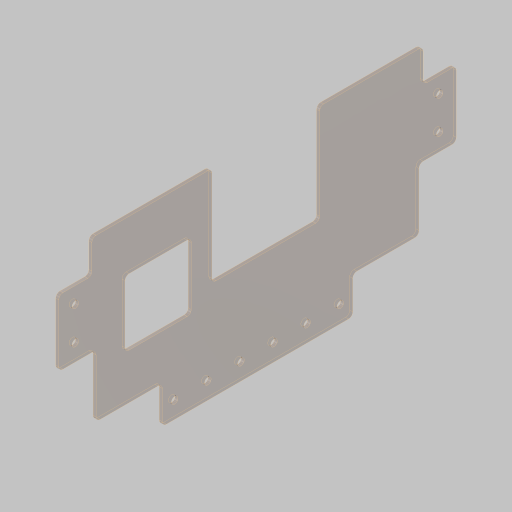
# Autodesk Inventor part: DB1-025
Saved by Autodesk Inventor 2023.5 (Build 275446000, 446)
## iProperties
Created: 2025-03-10
Part Number: DB1-025
Material: Polycarbonate, Smoke
Document SubType Name: Modeling
Designer: brand
Density: 1.2 g/cm^3
Appearance: Polycarbonate - Smoked
Author: brand
Autodesk Inventor part; units mm, degrees
ref_plane "YZ Plane" through (0, 0, 0) normal (1, 0, 0) x (0, 1, 0)
ref_plane "XZ Plane" through (0, 0, 0) normal (0, 1, 0) x (-1, 0, 0)
ref_plane "XY Plane" through (0, 0, 0) normal (0, 0, 1) x (1, 0, 0)
sketch "Sketch1" plane through (0, 0, 0) normal (1, 0, 0) x (0, 1, 0)
  line L0 (76.2, 152.4) -> (-76.2, 152.4)
  line L1 (-76.2, 152.4) -> (-76.2, -152.4)
  line L2 (-76.2, -152.4) -> (76.2, -152.4)
  line L3 (76.2, -152.4) -> (76.2, 152.4)
  line L4 (76.2, 152.4) -> (-76.2, -152.4) construction
  line L5 (-76.2, 152.4) -> (76.2, -152.4) construction
  line L6 (38.1, 101.6) -> (-12.7, 101.6)
  line L7 (-12.7, 101.6) -> (-12.7, 50.8)
  line L8 (-12.7, 50.8) -> (38.1, 50.8)
  line L9 (38.1, 50.8) -> (38.1, 101.6)
  line L10 (38.1, 101.6) -> (-12.7, 50.8) construction
  line L11 (-12.7, 101.6) -> (38.1, 50.8) construction
  line L12 (76.2, 34.925) -> (0, 34.925)
  line L13 (0, 34.925) -> (0, -47.625)
  line L14 (0, -47.625) -> (76.2, -47.625)
  line L15 (76.2, -47.625) -> (76.2, 34.925)
  line L16 (76.2, 34.925) -> (0, -47.625) construction
  line L17 (0, 34.925) -> (76.2, -47.625) construction
  point P0 (0, 0)
  point P1 (12.7, 76.2)
  point P2 (38.1, -6.35)
  point P3 (76.2, -6.35)
  point P4 (76.2, 0)
  point P5 (76.2, -47.625)
  point P6 (0, 44.45)
  point P7 (31.75, 44.45)
  point P8 (76.2, 34.925)
  dimension "d0" = 152.4
  dimension "d1" = 304.8
  dimension "d2" = 50.8
  dimension "d3" = 88.9
  dimension "d4" = 76.2
  dimension "d39" = 76.2
  dimension "d40" = 82.55
  dimension "d41" = 146.05
  constraints: 36 end point, 8 midpoint, 6 parallel, 4 perpendicular, 3 horizontal, 1 collinear
  measures "d0" distance of L2.end L1.end
  measures "d1" distance of L1.end L0.end
  measures "d2" distance of L8.end L6.start
  measures "d3" distance from line of L1 point (12.7, 76.2)
  measures "d4" distance from line of point (12.7, 76.2) L0
  measures "d39" distance of L13.end L14.end
  measures "d40" distance between parallel lines of L14 L12
  measures "d41" distance from line of L2 point (38.1, -6.35)
extrude "Extrusion1" add sketch "Sketch1" along normal blind 2.286 contours L3 L12 L13 L14 L2 L1 L0
fillet "Fillet1" radius 3.175 8 edges at (1.143, 38.1, 50.8) (1.143, 38.1, 101.6) (1.143, -12.7, 101.6) (1.143, -12.7, 50.8) (1.143, 76.2, 152.4) (1.143, 76.2, -152.4) (1.143, -76.2, -152.4) (1.143, -76.2, 152.4)
sketch "Sketch2" plane through (2.286, 0, 0) normal (1, 0, 0) x (0, 0, -1)
  arc A0 (-152.4, -73.025) -> (-149.225, -76.2) centre (-149.225, -73.025) ccw construction
  line L0 (-152.4, -73.025) -> (-152.4, 73.025) construction
  arc A1 (-149.225, 76.2) -> (-152.4, 73.025) centre (-149.225, 73.025) ccw construction
  line L1 (-149.225, 76.2) -> (-34.925, 76.2) construction
  arc A2 (152.4, 73.025) -> (149.225, 76.2) centre (149.225, 73.025) ccw construction
  line L2 (152.4, 73.025) -> (152.4, -73.025) construction
  arc A3 (149.225, -76.2) -> (152.4, -73.025) centre (149.225, -73.025) ccw construction
  line L3 (149.225, -76.2) -> (-149.225, -76.2) construction
  line L4 (-34.925, 76.2) -> (-34.925, 0) projected
  line L5 (-34.925, 0) -> (47.625, 0) projected
  line L6 (47.625, 0) -> (47.625, 76.2) projected
  line L7 (47.625, 76.2) -> (149.225, 76.2) projected
  arc A4 (-53.975, -12.7) -> (-50.8, -9.525) centre (-53.975, -9.525) ccw projected
  line L8 (-50.8, -9.525) -> (-50.8, 34.925) projected
  arc A5 (-50.8, 34.925) -> (-53.975, 38.1) centre (-53.975, 34.925) ccw projected
  line L9 (-53.975, 38.1) -> (-98.425, 38.1) projected
  arc A6 (-98.425, 38.1) -> (-101.6, 34.925) centre (-98.425, 34.925) ccw projected
  line L10 (-101.6, 34.925) -> (-101.6, -9.525) projected
  arc A7 (-101.6, -9.525) -> (-98.425, -12.7) centre (-98.425, -9.525) ccw projected
  line L11 (-98.425, -12.7) -> (-53.975, -12.7) projected
  point P0 (0, 0)
  point P1 (-139.7, -63.5)
  point P2 (139.7, -63.5)
  point P3 (-139.7, -38.1)
  point P4 (139.7, -38.1)
  point P5 (-139.7, -12.7)
  point P6 (139.7, -12.7)
  point P7 (-139.7, 12.7)
  point P8 (139.7, 12.7)
  point P9 (-139.7, 38.1)
  point P10 (139.7, 38.1)
  point P11 (-139.7, 63.5)
  point P12 (139.7, 63.5)
  point P13 (-114.3, -63.5)
  point P14 (-88.9, -63.5)
  point P15 (-63.5, -63.5)
  point P16 (-38.1, -63.5)
  point P17 (-12.7, -63.5)
  point P18 (12.7, -63.5)
  point P19 (38.1, -63.5)
  point P20 (63.5, -63.5)
  point P21 (88.9, -63.5)
  point P22 (114.3, -63.5)
  point P23 (139.7, -63.5)
  dimension "d8" = 12.7
  dimension "d9" = 12.7
  dimension "d10" = 12.7
  dimension "d13" = 25.4
  dimension "d34" = 25.4
  constraints: 1 horizontal, 1 horizontal alignment, 1 vertical, 21 other
  measures "d8" distance from line of L0 point (-139.7, -63.5)
  measures "d9" distance from line of L2 point (139.7, -63.5)
  measures "d10" distance from line of L3 point (139.7, -63.5)
  measures "d13" distance of point (-139.7, -63.5) point (-139.7, -38.1)
  measures "d34" distance of point (-139.7, -63.5) point (-114.3, -63.5)
hole "Hole1" at (2.286, -63.5, 139.7) at (2.286, -63.5, -139.7) at (2.286, -38.1, 139.7) at (2.286, -38.1, -139.7) at (2.286, -12.7, 139.7) at (2.286, -12.7, -139.7) at (2.286, 12.7, 139.7) at (2.286, 12.7, -139.7) at (2.286, 38.1, 139.7) at (2.286, 38.1, -139.7) at (2.286, 63.5, 139.7) at (2.286, 63.5, -139.7) at (2.286, -63.5, 88.9) at (2.286, -63.5, 63.5) at (2.286, -63.5, 38.1) at (2.286, -63.5, 12.7) at (2.286, -63.5, -12.7) at (2.286, -63.5, -38.1) at (2.286, -63.5, -63.5) at (2.286, -63.5, -88.9) direction (-1, 0, 0) diameter 5.1054 end through all clearance for "Flat Head Machine Screw (82)" size "#10" standard "Ansi Unified Screw Threads"
sketch "Sketch3" plane through (2.286, 0, 0) normal (1, 0, 0) x (0, 0, -1)
  line L0 (-123.825, 0) -> (-152.4, 0)
  line L1 (-152.4, 0) -> (-152.4, -76.2)
  line L2 (-152.4, -76.2) -> (-123.825, -76.2)
  line L3 (-123.825, -76.2) -> (-123.825, 0)
  line L4 (-123.825, 0) -> (-152.4, -76.2) construction
  line L5 (-152.4, 0) -> (-123.825, -76.2) construction
  circle A0 centre (-139.7, 63.5) radius 2.5527 construction
  circle A1 centre (-139.7, 38.1) radius 2.5527 construction
  circle A2 centre (-139.7, 12.7) radius 2.5527 construction
  circle A3 centre (-139.7, -12.7) radius 2.5527 construction
  circle A4 centre (-139.7, -38.1) radius 2.5527 construction
  circle A5 centre (-139.7, -63.5) radius 2.5527 construction
  circle A6 centre (139.7, -63.5) radius 2.5527 construction
  circle A7 centre (139.7, -38.1) radius 2.5527 construction
  circle A8 centre (139.7, -12.7) radius 2.5527 construction
  circle A9 centre (139.7, 12.7) radius 2.5527 construction
  circle A10 centre (139.7, 38.1) radius 2.5527 construction
  circle A11 centre (139.7, 63.5) radius 2.5527 construction
  arc A12 (-152.4, -73.025) -> (-149.225, -76.2) centre (-149.225, -73.025) ccw construction
  line L6 (-152.4, -73.025) -> (-152.4, 73.025) construction
  arc A13 (-149.225, 76.2) -> (-152.4, 73.025) centre (-149.225, 73.025) ccw construction
  line L7 (-149.225, 76.2) -> (-34.925, 76.2) construction
  arc A14 (152.4, 73.025) -> (149.225, 76.2) centre (149.225, 73.025) ccw construction
  line L8 (152.4, 73.025) -> (152.4, -73.025) construction
  arc A15 (149.225, -76.2) -> (152.4, -73.025) centre (149.225, -73.025) ccw construction
  line L9 (149.225, -76.2) -> (-149.225, -76.2) construction
  line L10 (-149.225, -76.2) -> (149.225, -76.2) construction
  line L11 (149.225, 76.2) -> (-149.225, 76.2) construction
  line L12 (0, 76.2) -> (0, -76.2) construction
  line L13 (-149.225, -76.2) -> (149.225, -76.2) construction
  line L14 (-152.4, -47.625) -> (-73.025, -47.625)
  line L15 (-73.025, -47.625) -> (-73.025, -76.2)
  line L16 (-73.025, -76.2) -> (-152.4, -76.2)
  line L17 (-152.4, -76.2) -> (-152.4, -47.625)
  line L18 (-152.4, -47.625) -> (-73.025, -76.2) construction
  line L19 (-73.025, -47.625) -> (-152.4, -76.2) construction
  line L20 (123.825, 0) -> (152.4, 0)
  line L21 (152.4, 0) -> (152.4, -76.2)
  line L22 (152.4, -76.2) -> (123.825, -76.2)
  line L23 (123.825, -76.2) -> (123.825, 0)
  line L24 (123.825, 0) -> (152.4, -76.2) construction
  line L25 (152.4, 0) -> (123.825, -76.2) construction
  circle A16 centre (139.7, -12.7) radius 2.5527 construction
  circle A17 centre (139.7, -38.1) radius 2.5527 construction
  circle A18 centre (139.7, -63.5) radius 2.5527 construction
  arc A19 (149.225, -76.2) -> (152.4, -73.025) centre (149.225, -73.025) ccw construction
  arc A20 (98.425, -25.4) -> (101.6, -22.225) centre (98.425, -22.225) ccw construction
  line L26 (152.4, -47.625) -> (73.025, -47.625)
  line L27 (73.025, -47.625) -> (73.025, -76.2)
  line L28 (73.025, -76.2) -> (152.4, -76.2)
  line L29 (152.4, -76.2) -> (152.4, -47.625)
  line L30 (152.4, -47.625) -> (73.025, -76.2) construction
  line L31 (73.025, -47.625) -> (152.4, -76.2) construction
  circle A21 centre (63.5, -63.5) radius 2.5527 projected
  circle A22 centre (12.7, -63.5) radius 2.5527 projected
  circle A23 centre (-38.1, -63.5) radius 2.5527 projected
  circle A24 centre (-88.9, -63.5) radius 2.5527 projected
  circle A25 centre (-63.5, -63.5) radius 2.5527 projected
  circle A26 centre (-12.7, -63.5) radius 2.5527 projected
  circle A27 centre (38.1, -63.5) radius 2.5527 projected
  circle A28 centre (88.9, -63.5) radius 2.5527 projected
  line L32 (-34.925, 76.2) -> (-34.925, 0) projected
  line L33 (-34.925, 0) -> (47.625, 0) projected
  line L34 (47.625, 0) -> (47.625, 76.2) projected
  line L35 (47.625, 76.2) -> (149.225, 76.2) projected
  arc A29 (-53.975, -12.7) -> (-50.8, -9.525) centre (-53.975, -9.525) ccw projected
  line L36 (-50.8, -9.525) -> (-50.8, 34.925) projected
  arc A30 (-50.8, 34.925) -> (-53.975, 38.1) centre (-53.975, 34.925) ccw projected
  line L37 (-53.975, 38.1) -> (-98.425, 38.1) projected
  arc A31 (-98.425, 38.1) -> (-101.6, 34.925) centre (-98.425, 34.925) ccw projected
  line L38 (-101.6, 34.925) -> (-101.6, -9.525) projected
  arc A32 (-101.6, -9.525) -> (-98.425, -12.7) centre (-98.425, -9.525) ccw projected
  line L39 (-98.425, -12.7) -> (-53.975, -12.7) projected
  line L40 (-127, 50.8) -> (-152.4, 50.8)
  line L41 (-152.4, 50.8) -> (-152.4, 76.2)
  line L42 (-152.4, 76.2) -> (-127, 76.2)
  line L43 (-127, 76.2) -> (-127, 50.8)
  circle A33 centre (139.7, 63.5) radius 2.5527 construction
  arc A34 (152.4, 73.025) -> (149.225, 76.2) centre (149.225, 73.025) ccw construction
  line L44 (127, 50.8) -> (152.4, 50.8)
  line L45 (152.4, 50.8) -> (152.4, 76.2)
  line L46 (152.4, 76.2) -> (127, 76.2)
  line L47 (127, 76.2) -> (127, 50.8)
  point P0 (0, 0)
  point P1 (-138.1125, -38.1)
  point P2 (-101.6, -22.225)
  point P3 (-98.425, -25.4)
  point P4 (-98.425, -22.225)
  point P5 (-112.7125, -61.9125)
  point P6 (138.1125, -38.1)
  point P7 (112.7125, -61.9125)
  point P8 (123.825, -47.625)
  point P9 (-123.825, -47.625)
  dimension "d25" = 28.575
  dimension "d26" = 76.2
  dimension "d27" = 28.575
  dimension "d28" = 79.375
  dimension "d42" = 25.4
  constraints: 66 end point, 23 symmetric about line, 7 centre point, 6 collinear, 6 midpoint, 6 parallel, 6 point on circle, 4 perpendicular, 3 horizontal, 6 other
  measures "d25" distance of L0.start L0.end
  measures "d26" distance of L0.end L1.end
  measures "d27" distance of L16.end L14.start
  measures "d28" distance of L15.end L16.end
  measures "d42" distance of L42.end L40.start
extrude "Extrusion2" cut sketch "Sketch3" against normal through all contours L3 L14 L1 L0 | L14 L15 L16 L3 | L3 L2 L1 L14 | L20 L21 L26 L23 | L26 L21 L22 L23 | L23 L28 L27 L26 | A24 | A28 | L35 L46 L45 L44 L47 | L40 L41 L42 L43
fillet "Fillet2" radius 3.175 20 edges at (1.143, 0, 152.4) (1.143, 0, 123.825) (1.143, -47.625, 123.825) (1.143, -47.625, 73.025) (1.143, -76.2, 73.025) (1.143, -76.2, -73.025) (1.143, -47.625, -73.025) (1.143, -47.625, -123.825) (1.143, 0, -123.825) (1.143, 0, -152.4) (1.143, 0, 34.925) (1.143, 0, -47.625) (1.143, 76.2, -47.625) (1.143, 76.2, 34.925) (1.143, 50.8, 127) (1.143, 76.2, 127) (1.143, 50.8, 152.4) (1.143, 76.2, -127) (1.143, 50.8, -127) (1.143, 50.8, -152.4)
equation "\"d9\" = d8"
equation "\"d10\" = d8"
body "Solid1"
